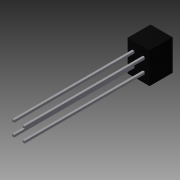
# Autodesk Inventor part: LineSensor
Saved by Autodesk Inventor 2015 (Build 190159000, 159)
## iProperties
Created: 2017-01-31
Part Number: LineSensor
Material: Generic
Document SubType Name: Modeling
Designer: Ernest
Density: 1 g/cm^3
Appearance: Default
Author: Ernest
Autodesk Inventor part; units mm, degrees
ref_plane "YZ Plane" through (0, 0, 0) normal (1, 0, 0) x (0, 1, 0)
ref_plane "XZ Plane" through (0, 0, 0) normal (0, 1, 0) x (-1, 0, 0)
ref_plane "XY Plane" through (0, 0, 0) normal (0, 0, 1) x (1, 0, 0)
sketch "Sketch1" plane through (0, 0, 0) normal (0, 1, 0) x (-1, 0, 0)
  line L0 (0, 0) -> (4.4, 0)
  line L1 (4.4, 0) -> (4.4, -6.16)
  line L2 (4.4, -6.16) -> (0, -6.16)
  line L3 (0, -6.16) -> (0, 0)
  dimension "d0" = 6.16
  dimension "d1" = 4.4
  constraints: 8 end point, 2 parallel, 1 horizontal, 1 perpendicular
  measures "d0" distance of L0.end L1.end
  measures "d1" distance of L1.end L2.end
extrude "Extrusion1" add sketch "Sketch1" along normal blind 4.6
sketch "Sketch2" plane through (0, 4.6, 0) normal (0, 1, 0) x (1, 0, 0)
  line L0 (-3.9333, 1.23) -> (-2.4333, 1.23)
  line L1 (-2.4333, 1.23) -> (-2.4333, 4.93)
  line L2 (-2.4333, 4.93) -> (-3.9333, 4.93)
  line L3 (-3.9333, 4.93) -> (-3.9333, 1.23)
  line L4 (-1.9667, 1.23) -> (-0.4667, 1.23)
  line L5 (-0.4667, 1.23) -> (-0.4667, 4.93)
  line L6 (-0.4667, 4.93) -> (-1.9667, 4.93)
  line L7 (-1.9667, 4.93) -> (-1.9667, 1.23)
  line L8 (-4.4, 0) -> (0, 0) projected
  line L9 (0, 0) -> (0, 6.16) projected
  line L10 (0, 6.16) -> (-4.4, 6.16) projected
  line L11 (-4.4, 6.16) -> (-4.4, 0) projected
  dimension "d4" = 3.7
  dimension "d5" = 1.5
  dimension "d6" = 4.4
  dimension "d7" = 0.4667
  dimension "d8" = 0.4667
  dimension "d9" = 6.16
  dimension "d10" = 1.23
  constraints: 16 end point, 4 parallel, 2 horizontal, 2 perpendicular, 2 point on line, 1 collinear
  measures "d4" distance of L2.end L0.start
  measures "d5" distance of L1.end L2.end
  measures "d6" distance of L9.end L10.end
  measures "d7" distance between parallel lines of L11 L3
  measures "d8" distance between parallel lines of L9 L5
  measures "d9" distance of L8.end L9.end
  measures "d10" distance between parallel lines of L10 L6
extrude "Extrusion2" cut sketch "Sketch2" against normal blind 0.05 contours L3 L2 L1 L0 | L7 L6 L5 L4
sketch "Sketch4" plane through (0, 0, 0) normal (0, -1, 0) x (1, 0, 0)
  line L0 (-3.45, -1.58) -> (-3.05, -1.58)
  line L1 (-3.05, -1.58) -> (-3.05, -2.03)
  line L2 (-3.05, -2.03) -> (-3.45, -2.03)
  line L3 (-3.45, -2.03) -> (-3.45, -1.58)
  line L4 (-1.35, -1.58) -> (-0.95, -1.58)
  line L5 (-0.95, -1.58) -> (-0.95, -2.03)
  line L6 (-0.95, -2.03) -> (-1.35, -2.03)
  line L7 (-1.35, -2.03) -> (-1.35, -1.58)
  line L8 (-3.45, -4.13) -> (-3.05, -4.13)
  line L9 (-3.05, -4.13) -> (-3.05, -4.58)
  line L10 (-3.05, -4.58) -> (-3.45, -4.58)
  line L11 (-3.45, -4.58) -> (-3.45, -4.13)
  line L12 (-1.35, -4.13) -> (-0.95, -4.13)
  line L13 (-0.95, -4.13) -> (-0.95, -4.58)
  line L14 (-0.95, -4.58) -> (-1.35, -4.58)
  line L15 (-1.35, -4.58) -> (-1.35, -4.13)
  line L16 (0, 0) -> (-4.4, 0) projected
  line L17 (-4.4, 0) -> (-4.4, -6.16) projected
  line L18 (-4.4, -6.16) -> (0, -6.16) projected
  line L19 (0, -6.16) -> (0, 0) projected
  dimension "d13" = 0.45
  dimension "d14" = 0.4
  dimension "d15" = 2.5
  dimension "d16" = 3
  dimension "d17" = 4.4
  dimension "d18" = 6.16
  dimension "d19" = 1.58
  dimension "d20" = 0.95
  constraints: 32 end point, 8 parallel, 7 collinear, 4 horizontal, 4 perpendicular, 3 point on line
  measures "d13" distance of L2.end L0.start
  measures "d14" distance of L0.start L0.end
  measures "d15" distance between parallel lines of L5 L3
  measures "d16" distance between parallel lines of L14 L4
  measures "d17" distance of L16.start L16.end
  measures "d18" distance of L16.end L17.end
  measures "d19" distance between parallel lines of L16 L4
  measures "d20" distance between parallel lines of L17 L3
extrude "Extrusion3" add sketch "Sketch4" along normal blind 24 contours L0 L1 L2 L3 | L4 L5 L6 L7 | L8 L9 L10 L11 | L12 L13 L14 L15
equation "\"d7\" = -0.666667 * d5 + 0.333333 * d6"
equation "\"d8\" = d7"
equation "\"d10\" = -0.5 * d4 + 0.5 * d9"
equation "\"d19\" = -0.5 * d16 + 0.5 * d18"
equation "\"d20\" = -0.5 * d15 + 0.5 * d17"
body "Solid1"
